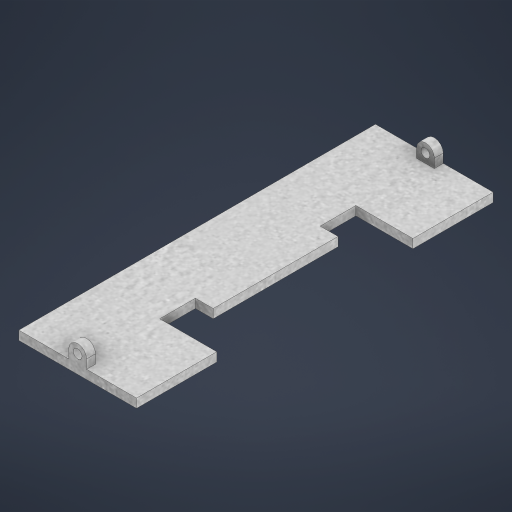
# Autodesk Inventor part: FP V2 Mounting Claw
Saved by Autodesk Inventor 2023.6 (Build 276521000, 521)
## iProperties
Created: 2026-02-22
Part Number: FP V2 Mounting Claw
Material: Generic
Document SubType Name: Modeling
Designer: user
Density: 1 g/cm^3
Appearance: Flat - Polished Gray
Author: user
Autodesk Inventor part; units mm, degrees
ref_plane "YZ Plane" through (0, 0, 0) normal (1, 0, 0) x (0, 1, 0)
ref_plane "XZ Plane" through (0, 0, 0) normal (0, 1, 0) x (-1, 0, 0)
sketch "Sketch1" plane through (0, 0, 0) normal (0, 1, 0) x (-1, 0, 0)
  line L0 (11, 55) -> (-11, 55)
  line L1 (-11, 55) -> (-11, -55)
  line L2 (-11, -55) -> (11, -55)
  line L3 (11, -55) -> (11, 55)
  line L4 (11, 55) -> (-11, -55) construction
  line L5 (-11, 55) -> (11, -55) construction
  line L6 (55, 100) -> (-55, 100)
  line L7 (-55, 100) -> (-55, -100)
  line L8 (-55, -100) -> (55, -100)
  line L9 (55, -100) -> (55, 100)
  line L10 (55, 100) -> (-55, -100) construction
  line L11 (-55, 100) -> (55, -100) construction
  line L12 (55, 100) -> (7.4, 100)
  line L13 (7.4, 100) -> (7.4, 46.4)
  line L14 (7.4, 46.4) -> (55, 46.4)
  line L15 (55, 46.4) -> (55, 100)
  line L16 (55, 0) -> (11, 0)
  circle A0 centre (33, 0) radius 4
  line L17 (-11, -55) -> (-11, -100)
  circle A1 centre (0, -75) radius 5
  point P0 (0, 0)
  dimension "d0" = 22
  dimension "d1" = 110
  dimension "d2" = 200
  dimension "d3" = 110
  dimension "d6" = 53.6
  dimension "d7" = 47.6
  dimension "d12" = 8
  dimension "d17" = 10
  dimension "d20" = 20
  constraints: 36 end point, 7 midpoint, 6 parallel, 4 perpendicular, 3 horizontal, 2 centre point, 1 point on line
  measures "d0" distance between parallel lines of L1 L3
  measures "d1" distance between parallel lines of L2 L0
  measures "d2" distance between parallel lines of L8 L6
  measures "d3" distance between parallel lines of L7 L9
  measures "d6" distance of L12.end L13.end
  measures "d7" distance of L13.end L14.end
  measures "d12" diameter of A0
  measures "d17" diameter of A1
  measures "d20" distance from line of L2 A1.centre
extrude "Extrusion1" add sketch "Sketch1" along normal blind 5 contours L0 L13 L6 L9 L14 L3 | L0 L1 L17 L8 L7 L6 L13 | L14 L9 L16 A0 L3 | L16 A0 L9 L8 L17 L2 L3 | A0 L16 | L16 A0 | A1
sketch "Sketch3" plane through (0, 5, 0) normal (0, 1, 0) x (1, 0, 0)
  line L0 (11, 55) -> (11, -55) projected
  line L1 (11, -55) -> (11, -100)
  line L2 (-55, -100) -> (55, -100) projected
  line L3 (-11, 55) -> (11, 55) projected
  line L4 (11, 55) -> (11, 100)
  line L5 (55, 100) -> (-55, 100) projected
  line L6 (55, -100) -> (55, 100) projected
  point P0 (0, 0)
  constraints: 4 end point, 3 point on line, 1 vertical
extrude "Extrusion3" cut sketch "Sketch3" against normal through all
sketch "Sketch4" plane through (0, 5, 0) normal (0, 1, 0) x (1, 0, 0)
  line L0 (-11, -55) -> (-11, 55) projected
  line L1 (-11, -55) -> (-21, -55)
  line L2 (-21, -55) -> (-21, -35)
  line L3 (-21, -35) -> (-11, -35)
  point P0 (0, 0)
  dimension "d21" = 10
  dimension "d22" = 20
  constraints: 6 end point, 2 perpendicular, 1 horizontal, 1 point on line
  measures "d21" distance of L0.start L1.end
  measures "d22" distance of L1.end L2.end
extrude "Extrusion6" cut sketch "Sketch4" against normal through all
mirror "Mirror1" about plane through (0, 0, 0) normal (0, 0, 1) of "Extrusion6"
sketch "Sketch5" plane through (-55, 0, 100) normal (0, 0, 1) x (1, 0, 0)
  circle A0 centre (33, 10) radius 2.5
  circle A1 centre (33, 10) radius 5
  line L0 (66, 0) -> (66, 5) projected
  line L1 (0, 5) -> (66, 5) projected
  line L2 (0, 0) -> (0, 5) projected
  line L3 (0, 0) -> (66, 0) projected
  line L4 (0, 5) -> (66, 5) projected
  line L5 (38, 10) -> (38, 5)
  line L6 (66, 5) -> (0, 5) projected
  line L7 (33, 0) -> (33, 5)
  line L8 (28, 10) -> (28, 5)
  point P0 (55, 0)
  point P1 (38, 5)
  point P2 (33, 5)
  point P3 (28, 5)
  dimension "d25" = 5
  dimension "d26" = 10
  constraints: 6 end point, 3 midpoint, 3 point on circle, 3 tangent, 2 centre point, 2 perpendicular, 2 point on line, 1 coincident
  measures "d25" diameter of A0
  measures "d26" diameter of A1
extrude "Extrusion7" add sketch "Sketch5" against normal blind 5 contours A1 | L5 L1 A1 | A1 L1 L8
ref_plane "Work Plane2" through (-55, 0, 0) normal (0, 0, 1) x (1, 0, 0)
mirror "Mirror4" about plane through (-55, 0, 0) normal (0, 0, 1) of "Extrusion7"
body "Solid1"
